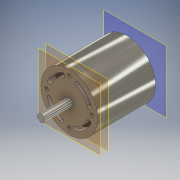
# Autodesk Inventor part: motor2
Saved by Autodesk Inventor 2018 (Build 220112000, 112)
## iProperties
Created: 2017-06-05
Part Number: motor2
Material: Generic
Document SubType Name: Modeling
Designer: Zadeka
Density: 1 g/cm^3
Appearance: Default
Author: Zadeka
Autodesk Inventor part; units mm, degrees
ref_plane "YZ Plane" through (0, 0, 0) normal (1, 0, 0) x (0, 1, 0)
ref_plane "XZ Plane" through (0, 0, 0) normal (0, 1, 0) x (-1, 0, 0)
ref_plane "XY Plane" through (0, 0, 0) normal (0, 0, 1) x (1, 0, 0)
sketch "Sketch1" plane through (0, 0, 0) normal (0, 1, 0) x (-1, 0, 0)
  circle A0 centre (0, 0) radius 31.5
  dimension "d0" = 63
  constraints: 1 centre point, 1 coincident
  measures "d0" diameter of A0
extrude "Extrusion1" add sketch "Sketch1" along normal blind 55
ref_plane "Work Plane1" through (0, 64, 0) normal (0, 1, 0) x (1, 0, 0)
sketch "Sketch2" plane through (0, 64, 0) normal (0, 1, 0) x (1, 0, 0)
  circle A0 centre (0, 0) radius 10
  dimension "d4" = 20
  constraints: 1 centre point, 1 coincident
  measures "d4" diameter of A0
loft "Loft1" add profiles "Sketch2" section 1 edges at (31.5, 55, 0)
sketch "Sketch3" plane through (0, 64, 0) normal (0, 1, 0) x (1, 0, 0)
  circle A0 centre (0, 0) radius 10
  constraints: 1 centre point, 1 coincident
extrude "Extrusion2" add sketch "Sketch3" along normal blind 2
ref_plane "Work Plane2" through (0, 66, 0) normal (0, 1, 0) x (1, 0, 0)
sketch "Sketch4" plane through (0, 66, 0) normal (0, 1, 0) x (1, 0, 0)
  circle A0 centre (0, 0) radius 5
  dimension "d12" = 10
  constraints: 1 centre point, 1 coincident
  measures "d12" diameter of A0
extrude "Extrusion3" add sketch "Sketch4" along normal blind 2
ref_plane "Work Plane3" through (0, -0.5, 0) normal (0, -1, 0) x (1, 0, 0)
sketch "Sketch5" plane through (0, 0, 0) normal (0, -1, 0) x (1, 0, 0)
  circle A0 centre (0, 0) radius 10 projected
  circle A1 centre (0, 0) radius 31.5
  dimension "d16" = 63
  constraints: 1 centre point, 1 coincident
  measures "d16" diameter of A1
extrude "Extrusion4" add sketch "Sketch5" along normal blind 9 contours A0 | A1
ref_plane "Work Plane4" through (0, -9, 0) normal (0, -1, 0) x (1, 0, 0)
sketch "Sketch6" plane through (0, -9, 0) normal (0, -1, 0) x (1, 0, 0)
  circle A0 centre (0, 0) radius 10 projected
  circle A1 centre (0, 0) radius 4
  dimension "d20" = 8
  constraints: 1 centre point, 1 coincident
  measures "d20" diameter of A1
extrude "Extrusion5" add sketch "Sketch6" along normal blind 31.25 contours A1
sketch "Sketch7" plane through (0, 64, 0) normal (0, 1, 0) x (1, 0, 0)
  line L0 (0, 0) -> (-31.5, 0)
  circle A0 centre (0, 0) radius 31.5 projected
  line L1 (0, 0) -> (0, -31.5)
  line L2 (0, -15.75) -> (-15.75, 0)
  line L3 (-7.875, -7.875) -> (-18.4816, -18.4816)
  line L4 (-22.9102, -14.053) -> (-14.053, -22.9102)
  line L5 (-10.6776, -21.8882) -> (-8.4633, -10.8167)
  line L6 (-21.8882, -10.6776) -> (-10.8167, -8.4633)
  arc A1 (-21.8882, -10.6776) -> (-22.9102, -14.053) centre (-21.496, -12.6388) ccw
  arc A2 (-14.053, -22.9102) -> (-10.6776, -21.8882) centre (-12.6388, -21.496) ccw
  arc A3 (-8.4633, -10.8167) -> (-10.8167, -8.4633) centre (-10.4245, -10.4245) ccw
  line L7 (-14.7601, -23.6173) -> (-23.6173, -14.7601)
  arc A4 (-22.0843, -9.6971) -> (-23.6173, -14.7601) centre (-21.496, -12.6388) ccw
  line L8 (-22.0843, -9.6971) -> (-11.0129, -7.4828)
  arc A5 (-7.4828, -11.0129) -> (-11.0129, -7.4828) centre (-10.4245, -10.4245) ccw
  line L9 (-7.4828, -11.0129) -> (-9.6971, -22.0843)
  arc A6 (-14.7601, -23.6173) -> (-9.6971, -22.0843) centre (-12.6388, -21.496) ccw
  line L10 (17.9003, -21.3359) -> (6.7396, -27.0225)
  arc A7 (17.9003, -21.3359) -> (18.0069, -16.0469) centre (16.5383, -18.6628) ccw
  line L11 (8.1615, -10.5197) -> (18.0069, -16.0469)
  arc A8 (8.1615, -10.5197) -> (3.7134, -12.7862) centre (6.6929, -13.1356) ccw
  line L12 (2.398, -24) -> (3.7134, -12.7862)
  arc A9 (2.398, -24) -> (6.7396, -27.0225) centre (5.3776, -24.3495) ccw
  line L13 (25.8231, 10.431) -> (27.7826, -1.9407)
  arc A10 (25.8231, 10.431) -> (20.8259, 12.1668) centre (22.86, 9.9617) ccw
  line L14 (12.5269, 4.5113) -> (20.8259, 12.1668)
  arc A11 (12.5269, 4.5113) -> (13.3078, -0.4195) centre (14.561, 2.3062) ccw
  line L15 (23.5664, -5.1358) -> (13.3078, -0.4195)
  arc A12 (23.5664, -5.1358) -> (27.7826, -1.9407) centre (24.8195, -2.41) ccw
  line L16 (-1.9407, 27.7826) -> (10.431, 25.8231)
  arc A13 (-1.9407, 27.7826) -> (-5.1358, 23.5664) centre (-2.41, 24.8195) ccw
  line L17 (-0.4195, 13.3078) -> (-5.1358, 23.5664)
  arc A14 (-0.4195, 13.3078) -> (4.5113, 12.5269) centre (2.3062, 14.561) ccw
  line L18 (12.1668, 20.8259) -> (4.5113, 12.5269)
  arc A15 (12.1668, 20.8259) -> (10.431, 25.8231) centre (9.9617, 22.86) ccw
  line L19 (-27.0225, 6.7396) -> (-21.3359, 17.9003)
  arc A16 (-27.0225, 6.7396) -> (-24, 2.398) centre (-24.3495, 5.3776) ccw
  line L20 (-12.7862, 3.7134) -> (-24, 2.398)
  arc A17 (-12.7862, 3.7134) -> (-10.5197, 8.1615) centre (-13.1356, 6.6929) ccw
  line L21 (-16.0469, 18.0069) -> (-10.5197, 8.1615)
  arc A18 (-16.0469, 18.0069) -> (-21.3359, 17.9003) centre (-18.6628, 16.5383) ccw
  point P0 (-25.5527, -11.4105)
  point P1 (-11.4105, -25.5527)
  dimension "d23" = 15
  dimension "d24" = 10
  dimension "d25" = 20
  dimension "d26" = 2
  dimension "d27" = 1
  dimension "d30" = 360
  constraints: 44 end point, 38 point on circle, 18 centre point, 6 point on line, 6 tangent, 3 midpoint, 2 equal radius, 2 perpendicular, 1 horizontal, 1 vertical, 81 other
  measures "d23" distance of L3.start L3.end
  measures "d24" distance of L3.end point (-25.553, -11.411)
  measures "d25" distance of point (-25.553, -11.411) point (-11.411, -25.553)
  measures "d26" radius of A1
  measures "d27" distance between parallel lines of L4 L7
extrude "Extrusion6" cut sketch "Sketch7" against normal blind 9 contours A3 L5 A2 L4 L3 | L3 L4 A1 L6 A3 | L7 A4 L8 A5 L9 A6 | L10 A9 L12 A8 L11 A7 | L13 A12 L15 A11 L14 A10 | L16 A15 L18 A14 L17 A13 | L19 A18 L21 A17 L20 A16
sketch "Sketch8" plane through (0, -9, 0) normal (0, -1, 0) x (1, 0, 0)
  line L0 (0, 0) -> (0, -25)
  circle A0 centre (0, -25) radius 2
  circle A1 centre (25, 0) radius 2
  circle A2 centre (0, 25) radius 2
  circle A3 centre (-25, 0) radius 2
  circle A4 centre (0, 0) radius 5 projected
  circle A5 centre (0, 0) radius 31.5 projected
  circle A6 centre (0, 0) radius 4 projected
  arc A7 (6.4072, -20.0682) -> (8.6161, -23.8742) centre (7.0925, -22.2145) ccw
  arc A8 (23.2351, -10.194) -> (19.5995, -7.723) centre (21.6957, -8.5489) ccw
  arc A9 (7.0925, -24.4675) -> (23.2351, -10.194) centre (-2.6577, 2.8244) ccw
  arc A10 (6.4072, -20.0682) -> (19.5995, -7.723) centre (0, 0) ccw
  arc A11 (24.4675, 7.0925) -> (10.194, 23.2351) centre (-2.8244, -2.6577) ccw
  arc A12 (20.0682, 6.4072) -> (23.8742, 8.6161) centre (22.2145, 7.0925) ccw
  arc A13 (20.0682, 6.4072) -> (7.723, 19.5995) centre (0, 0) ccw
  arc A14 (10.194, 23.2351) -> (7.723, 19.5995) centre (8.5489, 21.6957) ccw
  arc A15 (-7.0925, 24.4675) -> (-23.2351, 10.194) centre (2.6577, -2.8244) ccw
  arc A16 (-6.4072, 20.0682) -> (-8.6161, 23.8742) centre (-7.0925, 22.2145) ccw
  arc A17 (-6.4072, 20.0682) -> (-19.5995, 7.723) centre (0, 0) ccw
  arc A18 (-23.2351, 10.194) -> (-19.5995, 7.723) centre (-21.6957, 8.5489) ccw
  arc A19 (-24.4675, -7.0925) -> (-10.194, -23.2351) centre (2.8244, 2.6577) ccw
  arc A20 (-20.0682, -6.4072) -> (-23.8742, -8.6161) centre (-22.2145, -7.0925) ccw
  arc A21 (-20.0682, -6.4072) -> (-7.723, -19.5995) centre (0, 0) ccw
  arc A22 (-10.194, -23.2351) -> (-7.723, -19.5995) centre (-8.5489, -21.6957) ccw
  dimension "d34" = 25
  dimension "d35" = 4
  dimension "d38" = 360
  dimension "d46" = 360
  constraints: 40 point on circle, 20 centre point, 2 end point, 1 coincident, 1 vertical, 62 other
  measures "d34" distance of L0.start L0.end
  measures "d35" diameter of A0
extrude "Extrusion7" cut sketch "Sketch8" against normal blind 9 contours A0 | A1 | A2 | A3 | A10 A8 A9 A7 | A12 A13 A14 A11 | A16 A17 A18 A15 | A20 A21 A22 A19
thread "Thread1" size "M4x0.7" class "6H" standard "ANSI Metric M Profile" full length
thread "Thread2" size "M4x0.7" class "6H" standard "ANSI Metric M Profile" full length
thread "Thread3" size "M4x0.7" class "6H" standard "ANSI Metric M Profile" full length
thread "Thread4" size "M4x0.7" class "6H" standard "ANSI Metric M Profile" full length
body "Solid1"
